Autodesk Inventor part; units mm, degrees
(part 2 of 2)
  line L340 (-1.9195, 5.2475) -> (-1.8042, 5.1384)
  line L341 (-2.0415, 5.3441) -> (-1.9195, 5.2475)
  line L342 (-2.1047, 5.3882) -> (-2.0415, 5.3441)
  line L343 (-2.1649, 5.4382) -> (-2.1047, 5.3882)
  line L344 (-2.2201, 5.4981) -> (-2.1649, 5.4382)
  line L345 (-2.2447, 5.5342) -> (-2.2201, 5.4981)
  line L346 (-2.2651, 5.5787) -> (-2.2447, 5.5342)
  line L347 (-2.2631, 5.6693) -> (-2.2651, 5.5787)
  line L348 (-1.9339, 6.464) -> (-2.2631, 5.6693)
  line L349 (-1.8713, 6.5294) -> (-1.9339, 6.464)
  line L350 (-1.8254, 6.5464) -> (-1.8713, 6.5294)
  line L351 (-1.7825, 6.5547) -> (-1.8254, 6.5464)
  line L352 (-1.7011, 6.5579) -> (-1.7825, 6.5547)
  line L353 (-1.6232, 6.5508) -> (-1.7011, 6.5579)
  line L354 (-1.5473, 6.5372) -> (-1.6232, 6.5508)
  line L355 (-1.3927, 6.5193) -> (-1.5473, 6.5372)
  line L356 (-1.2341, 6.5149) -> (-1.3927, 6.5193)
  line L357 (-1.0724, 6.5212) -> (-1.2341, 6.5149)
  line L358 (-0.9083, 6.5371) -> (-1.0724, 6.5212)
  line L359 (-0.7422, 6.5617) -> (-0.9083, 6.5371)
  line L360 (-0.5744, 6.5945) -> (-0.7422, 6.5617)
  line L361 (-0.4052, 6.6353) -> (-0.5744, 6.5945)
  line L362 (-0.2775, 6.671) -> (-0.4052, 6.6353)
  line L363 (-0.0892, 7.6173) -> (-0.2775, 6.671)
  line L364 (-0.1935, 7.6991) -> (-0.0892, 7.6173)
  line L365 (-0.3343, 7.8015) -> (-0.1935, 7.6991)
  line L366 (-0.4767, 7.8961) -> (-0.3343, 7.8015)
  line L367 (-0.6208, 7.9824) -> (-0.4767, 7.8961)
  line L368 (-0.7663, 8.0598) -> (-0.6208, 7.9824)
  line L369 (-0.9133, 8.1276) -> (-0.7663, 8.0598)
  line L370 (-1.0615, 8.1842) -> (-0.9133, 8.1276)
  line L371 (-1.2112, 8.2268) -> (-1.0615, 8.1842)
  line L372 (-1.2865, 8.2433) -> (-1.2112, 8.2268)
  line L373 (-1.3612, 8.2665) -> (-1.2865, 8.2433)
  line L374 (-1.4352, 8.3007) -> (-1.3612, 8.2665)
  line L375 (-1.4717, 8.3247) -> (-1.4352, 8.3007)
  line L376 (-1.5076, 8.358) -> (-1.4717, 8.3247)
  line L377 (-1.5404, 8.4424) -> (-1.5076, 8.358)
  line L378 (-1.5404, 9.3026) -> (-1.5404, 8.4424)
  line L379 (-1.5076, 9.387) -> (-1.5404, 9.3026)
  line L380 (-1.4717, 9.4203) -> (-1.5076, 9.387)
  line L381 (-1.4352, 9.4443) -> (-1.4717, 9.4203)
  line L382 (-1.3612, 9.4785) -> (-1.4352, 9.4443)
  line L383 (-1.2865, 9.5017) -> (-1.3612, 9.4785)
  line L384 (-1.2112, 9.5182) -> (-1.2865, 9.5017)
  line L385 (-1.0615, 9.5608) -> (-1.2112, 9.5182)
  line L386 (-0.9133, 9.6174) -> (-1.0615, 9.5608)
  line L387 (-0.7663, 9.6852) -> (-0.9133, 9.6174)
  line L388 (-0.6208, 9.7626) -> (-0.7663, 9.6852)
  line L389 (-0.4767, 9.8489) -> (-0.6208, 9.7626)
  line L390 (-0.3343, 9.9435) -> (-0.4767, 9.8489)
  line L391 (-0.1935, 10.0459) -> (-0.3343, 9.9435)
  line L392 (-0.0892, 10.1277) -> (-0.1935, 10.0459)
  line L393 (-0.2775, 11.074) -> (-0.0892, 10.1277)
  line L394 (-0.4052, 11.1097) -> (-0.2775, 11.074)
  line L395 (-0.5744, 11.1505) -> (-0.4052, 11.1097)
  line L396 (-0.7422, 11.1834) -> (-0.5744, 11.1505)
  line L397 (-0.9083, 11.208) -> (-0.7422, 11.1834)
  line L398 (-1.0724, 11.2238) -> (-0.9083, 11.208)
  line L399 (-1.2341, 11.2302) -> (-1.0724, 11.2238)
  line L400 (-1.3927, 11.2258) -> (-1.2341, 11.2302)
  line L401 (-1.5473, 11.2079) -> (-1.3927, 11.2258)
  line L402 (-1.6232, 11.1943) -> (-1.5473, 11.2079)
  line L403 (-1.7011, 11.1871) -> (-1.6232, 11.1943)
  line L404 (-1.7825, 11.1904) -> (-1.7011, 11.1871)
  line L405 (-1.8254, 11.1986) -> (-1.7825, 11.1904)
  line L406 (-1.8713, 11.2156) -> (-1.8254, 11.1986)
  line L407 (-1.9339, 11.281) -> (-1.8713, 11.2156)
  line L408 (-2.2631, 12.0757) -> (-1.9339, 11.281)
  line L409 (-2.2651, 12.1663) -> (-2.2631, 12.0757)
  line L410 (-2.2447, 12.2108) -> (-2.2651, 12.1663)
  line L411 (-2.2201, 12.247) -> (-2.2447, 12.2108)
  line L412 (-2.1649, 12.3068) -> (-2.2201, 12.247)
  line L413 (-2.1047, 12.3569) -> (-2.1649, 12.3068)
  line L414 (-2.0415, 12.4009) -> (-2.1047, 12.3569)
  line L415 (-1.9195, 12.4975) -> (-2.0415, 12.4009)
  line L416 (-1.8042, 12.6066) -> (-1.9195, 12.4975)
  line L417 (-1.6944, 12.7254) -> (-1.8042, 12.6066)
  line L418 (-1.5896, 12.8527) -> (-1.6944, 12.7254)
  line L419 (-1.4895, 12.9875) -> (-1.5896, 12.8527)
  line L420 (-1.3941, 13.1294) -> (-1.4895, 12.9875)
  line L421 (-1.3032, 13.2779) -> (-1.3941, 13.1294)
  line L422 (-1.2382, 13.3934) -> (-1.3032, 13.2779)
  line L423 (-1.7742, 14.1957) -> (-1.2382, 13.3934)
  line L424 (-1.9058, 14.1797) -> (-1.7742, 14.1957)
  line L425 (-2.0778, 14.1527) -> (-1.9058, 14.1797)
  line L426 (-2.2454, 14.1188) -> (-2.0778, 14.1527)
  line L427 (-2.4083, 14.078) -> (-2.2454, 14.1188)
  line L428 (-2.5659, 14.0298) -> (-2.4083, 14.078)
  line L429 (-2.7177, 13.9738) -> (-2.5659, 14.0298)
  line L430 (-2.8626, 13.909) -> (-2.7177, 13.9738)
  line L431 (-2.9986, 13.8333) -> (-2.8626, 13.909)
  line L432 (-3.0635, 13.7917) -> (-2.9986, 13.8333)
  line L433 (-3.1327, 13.7553) -> (-3.0635, 13.7917)
  line L434 (-3.2092, 13.7272) -> (-3.1327, 13.7553)
  line L435 (-3.2519, 13.7183) -> (-3.2092, 13.7272)
  line L436 (-3.3009, 13.7165) -> (-3.2519, 13.7183)
  line L437 (-3.3838, 13.753) -> (-3.3009, 13.7165)
  line L438 (-3.9921, 14.3612) -> (-3.3838, 13.753)
  line L439 (-4.0285, 14.4441) -> (-3.9921, 14.3612)
  line L440 (-4.0267, 14.4931) -> (-4.0285, 14.4441)
  line L441 (-4.0179, 14.5359) -> (-4.0267, 14.4931)
  line L442 (-3.9898, 14.6123) -> (-4.0179, 14.5359)
  line L443 (-3.9533, 14.6815) -> (-3.9898, 14.6123)
  line L444 (-3.9117, 14.7464) -> (-3.9533, 14.6815)
  line L445 (-3.836, 14.8824) -> (-3.9117, 14.7464)
  line L446 (-3.7712, 15.0273) -> (-3.836, 14.8824)
  line L447 (-3.7152, 15.1791) -> (-3.7712, 15.0273)
  line L448 (-3.6671, 15.3368) -> (-3.7152, 15.1791)
  line L449 (-3.6262, 15.4996) -> (-3.6671, 15.3368)
  line L450 (-3.5924, 15.6672) -> (-3.6262, 15.4996)
  line L451 (-3.5653, 15.8392) -> (-3.5924, 15.6672)
  line L452 (-3.5494, 15.9708) -> (-3.5653, 15.8392)
  line L453 (-4.3516, 16.5068) -> (-3.5494, 15.9708)
  line L454 (-4.4671, 16.4418) -> (-4.3516, 16.5068)
  line L455 (-4.6156, 16.351) -> (-4.4671, 16.4418)
  line L456 (-4.7575, 16.2555) -> (-4.6156, 16.351)
  line L457 (-4.8924, 16.1555) -> (-4.7575, 16.2555)
  line L458 (-5.0196, 16.0506) -> (-4.8924, 16.1555)
  line L459 (-5.1384, 15.9408) -> (-5.0196, 16.0506)
  line L460 (-5.2475, 15.8255) -> (-5.1384, 15.9408)
  line L461 (-5.3441, 15.7035) -> (-5.2475, 15.8255)
  line L462 (-5.3882, 15.6403) -> (-5.3441, 15.7035)
  line L463 (-5.4382, 15.5801) -> (-5.3882, 15.6403)
  line L464 (-5.4981, 15.5249) -> (-5.4382, 15.5801)
  line L465 (-5.5342, 15.5004) -> (-5.4981, 15.5249)
  line L466 (-5.5787, 15.4799) -> (-5.5342, 15.5004)
  line L467 (-5.6693, 15.4819) -> (-5.5787, 15.4799)
  line L468 (-6.464, 15.8111) -> (-5.6693, 15.4819)
  line L469 (-6.5294, 15.8737) -> (-6.464, 15.8111)
  line L470 (-6.5464, 15.9196) -> (-6.5294, 15.8737)
  line L471 (-6.5547, 15.9626) -> (-6.5464, 15.9196)
  line L472 (-6.5579, 16.0439) -> (-6.5547, 15.9626)
  line L473 (-6.5508, 16.1219) -> (-6.5579, 16.0439)
  line L474 (-6.5372, 16.1977) -> (-6.5508, 16.1219)
  line L475 (-6.5193, 16.3523) -> (-6.5372, 16.1977)
  line L476 (-6.5149, 16.511) -> (-6.5193, 16.3523)
  line L477 (-6.5212, 16.6726) -> (-6.5149, 16.511)
  line L478 (-6.5371, 16.8367) -> (-6.5212, 16.6726)
  line L479 (-6.5617, 17.0028) -> (-6.5371, 16.8367)
  line L480 (-6.5945, 17.1706) -> (-6.5617, 17.0028)
  line L481 (-6.6353, 17.3399) -> (-6.5945, 17.1706)
  line L482 (-6.671, 17.4675) -> (-6.6353, 17.3399)
  line L483 (-7.6173, 17.6558) -> (-6.671, 17.4675)
  line L484 (-7.6991, 17.5515) -> (-7.6173, 17.6558)
  line L485 (-7.8015, 17.4107) -> (-7.6991, 17.5515)
  line L486 (-7.8961, 17.2683) -> (-7.8015, 17.4107)
  line L487 (-7.9824, 17.1242) -> (-7.8961, 17.2683)
  line L488 (-8.0598, 16.9787) -> (-7.9824, 17.1242)
  line L489 (-8.1276, 16.8317) -> (-8.0598, 16.9787)
  line L490 (-8.1842, 16.6835) -> (-8.1276, 16.8317)
  line L491 (-8.2268, 16.5338) -> (-8.1842, 16.6835)
  line L492 (-8.2433, 16.4585) -> (-8.2268, 16.5338)
  line L493 (-8.2665, 16.3838) -> (-8.2433, 16.4585)
  line L494 (-8.3007, 16.3099) -> (-8.2665, 16.3838)
  line L495 (-8.3247, 16.2734) -> (-8.3007, 16.3099)
  line L496 (-8.358, 16.2375) -> (-8.3247, 16.2734)
  line L497 (-8.4424, 16.2046) -> (-8.358, 16.2375)
  line L498 (-9.3026, 16.2046) -> (-8.4424, 16.2046)
  line L499 (-9.387, 16.2375) -> (-9.3026, 16.2046)
  line L500 (-9.4203, 16.2734) -> (-9.387, 16.2375)
  line L501 (-9.4443, 16.3099) -> (-9.4203, 16.2734)
  line L502 (-9.4785, 16.3838) -> (-9.4443, 16.3099)
  line L503 (-9.5017, 16.4585) -> (-9.4785, 16.3838)
  line L504 (-9.5182, 16.5338) -> (-9.5017, 16.4585)
  line L505 (-9.5608, 16.6835) -> (-9.5182, 16.5338)
  line L506 (-9.6174, 16.8317) -> (-9.5608, 16.6835)
  line L507 (-9.6852, 16.9787) -> (-9.6174, 16.8317)
  line L508 (-9.7626, 17.1242) -> (-9.6852, 16.9787)
  line L509 (-9.8489, 17.2683) -> (-9.7626, 17.1242)
  line L510 (-9.9435, 17.4107) -> (-9.8489, 17.2683)
  line L511 (-10.0459, 17.5515) -> (-9.9435, 17.4107)
  line L512 (-10.1277, 17.6558) -> (-10.0459, 17.5515)
  line L513 (-11.074, 17.4675) -> (-10.1277, 17.6558)
  line L514 (-11.1097, 17.3399) -> (-11.074, 17.4675)
  line L515 (-11.1505, 17.1706) -> (-11.1097, 17.3399)
  line L516 (-11.1834, 17.0028) -> (-11.1505, 17.1706)
  line L517 (-7.2831, 7.0602) -> (-7.5453, 6.8602)
  line L518 (-7.0507, 7.294) -> (-7.2831, 7.0602)
  line L519 (-6.8523, 7.5573) -> (-7.0507, 7.294)
  line L520 (-6.6918, 7.8453) -> (-6.8523, 7.5573)
  line L521 (-6.047, 8.4605) -> (-6.6918, 7.8453)
  line L522 (-3.4326, 8.9806) -> (-6.047, 8.4605)
  line L523 (-2.9676, 8.5861) -> (-3.4326, 8.9806)
  line L524 (-3, 8.1922) -> (-2.9676, 8.5861)
  line L525 (-3.0586, 7.8013) -> (-3, 8.1922)
  line L526 (-3.1431, 7.4153) -> (-3.0586, 7.8013)
  line L527 (-3.2533, 7.0357) -> (-3.1431, 7.4153)
  line L528 (-3.3886, 6.6644) -> (-3.2533, 7.0357)
  line L529 (-3.5484, 6.3029) -> (-3.3886, 6.6644)
  line L530 (-3.732, 5.9529) -> (-3.5484, 6.3029)
  line L531 (-3.9385, 5.616) -> (-3.732, 5.9529)
  line L532 (-4.1671, 5.2936) -> (-3.9385, 5.616)
  line L533 (-4.4168, 4.9872) -> (-4.1671, 5.2936)
  line L534 (-4.6863, 4.6982) -> (-4.4168, 4.9872)
  line L535 (-4.9746, 4.4278) -> (-4.6863, 4.6982)
  line L536 (-5.2803, 4.1773) -> (-4.9746, 4.4278)
  line L537 (-5.602, 3.9478) -> (-5.2803, 4.1773)
  line L538 (-5.9384, 3.7402) -> (-5.602, 3.9478)
  line L539 (-6.2878, 3.5557) -> (-5.9384, 3.7402)
  line L540 (-6.6489, 3.3949) -> (-6.2878, 3.5557)
  line L541 (-7.0198, 3.2585) -> (-6.6489, 3.3949)
  line L542 (-7.3991, 3.1473) -> (-7.0198, 3.2585)
  line L543 (-7.7849, 3.0616) -> (-7.3991, 3.1473)
  line L544 (-8.1756, 3.0019) -> (-7.7849, 3.0616)
  line L545 (-8.5694, 2.9685) -> (-8.1756, 3.0019)
  line L546 (-8.9645, 2.9614) -> (-8.5694, 2.9685)
  line L547 (-9.3593, 2.9808) -> (-8.9645, 2.9614)
  line L548 (-9.6897, 3.4932) -> (-9.3593, 2.9808)
  line L549 (-8.8329, 6.0174) -> (-9.6897, 3.4932)
  line L550 (-8.1387, 6.5764) -> (-8.8329, 6.0174)
  line L551 (-7.8323, 6.698) -> (-8.1387, 6.5764)
  line L552 (-7.5453, 6.8602) -> (-7.8323, 6.698)
  line L553 (-12.7072, 4.3731) -> (-12.3979, 4.1269)
  line L554 (-12.9992, 4.6393) -> (-12.7072, 4.3731)
  line L555 (-13.2728, 4.9245) -> (-12.9992, 4.6393)
  line L556 (-13.5268, 5.2274) -> (-13.2728, 4.9245)
  line L557 (-13.7599, 5.5465) -> (-13.5268, 5.2274)
  line L558 (-13.9712, 5.8805) -> (-13.7599, 5.5465)
  line L559 (-14.1598, 6.2278) -> (-13.9712, 5.8805)
  line L560 (-14.3246, 6.587) -> (-14.1598, 6.2278)
  line L561 (-14.4652, 6.9564) -> (-14.3246, 6.587)
  line L562 (-14.5807, 7.3343) -> (-14.4652, 6.9564)
  line L563 (-14.6707, 7.7192) -> (-14.5807, 7.3343)
  line L564 (-14.7348, 8.1092) -> (-14.6707, 7.7192)
  line L565 (-14.7727, 8.5025) -> (-14.7348, 8.1092)
  line L566 (-14.7843, 8.8976) -> (-14.7727, 8.5025)
  line L567 (-14.7694, 9.2925) -> (-14.7843, 8.8976)
  line L568 (-14.7281, 9.6856) -> (-14.7694, 9.2925)
  line L569 (-14.6607, 10.075) -> (-14.7281, 9.6856)
  line L570 (-14.5674, 10.4591) -> (-14.6607, 10.075)
  line L571 (-14.4487, 10.836) -> (-14.5674, 10.4591)
  line L572 (-14.305, 11.2042) -> (-14.4487, 10.836)
  line L573 (-14.1371, 11.562) -> (-14.305, 11.2042)
  line L574 (-13.9457, 11.9077) -> (-14.1371, 11.562)
  line L575 (-13.7315, 12.2399) -> (-13.9457, 11.9077)
  line L576 (-13.1225, 12.2699) -> (-13.7315, 12.2399)
  line L577 (-11.3649, 10.2657) -> (-13.1225, 12.2699)
  line L578 (-11.2279, 9.3851) -> (-11.3649, 10.2657)
  line L579 (-11.2758, 9.0589) -> (-11.2279, 9.3851)
  line L580 (-11.2788, 8.7292) -> (-11.2758, 9.0589)
  line L581 (-11.2367, 8.4022) -> (-11.2788, 8.7292)
  line L582 (-11.1505, 8.084) -> (-11.2367, 8.4022)
  line L583 (-11.0216, 7.7806) -> (-11.1505, 8.084)
  line L584 (-10.8525, 7.4976) -> (-11.0216, 7.7806)
  line L585 (-10.642, 6.6316) -> (-10.8525, 7.4976)
  line L586 (-11.4989, 4.1074) -> (-10.642, 6.6316)
  line L587 (-12.073, 3.902) -> (-11.4989, 4.1074)
  line L588 (-12.3979, 4.1269) -> (-12.073, 3.902)
  circle A2 centre (-8.8725, 8.8725) radius 2.4105
  point P0 (0, 0)
  point P1 (-11.0215, 7.7805)
  point P2 (-8.1387, 6.5764)
  point P3 (-6.6918, 7.8453)
  point P4 (-7.2509, 10.6561)
  constraints: 1 coincident, 3 other
extrude "Выдавливание3" add sketch "Эскиз3" along normal blind 4 contours A1 L36 A0 L35 L34 L33 A2 L520 L519 L518 L517 L552 L551 L584 L583 L582 L581 L580 L579 L2 L1 L0 | L584 A2
